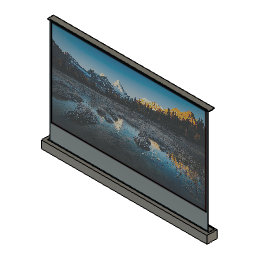
cabinet_model (Autodesk Fusion 360 archive; units mm, degrees)
design "Vividstorm S Pro 110"
Autodesk Fusion 360 part; units mm, degrees
sketch "Base sketch" plane through (0, 0, 0) normal (0, 0, 1) x (1, 0, 0)
  line L0 (0, 0) -> (2610, 0)
  line L1 (2610, 0) -> (2610, 160)
  line L2 (2610, 160) -> (0, 160)
  line L3 (0, 160) -> (0, 0)
  dimension "base_width" = 2610
  dimension "base_depth" = 160
  constraint horizontal L0
  constraint vertical L1
  constraint horizontal L2
  constraint vertical L3
  constraint coincident L0.start L3.end
  measures "base_width" distance of L0.start L0.end
  measures "base_depth" distance of L0.start L2.end
extrude "Extrude1" add sketch "Base sketch" along normal blind 120 makes body 1
sketch "Lid sketch" plane through (0, 0, 120) normal (0, 0, 1) x (-1, 0, 0)
  line L0 (0, -160) -> (0, 0)
  line L1 (0, 0) -> (-2610, 0)
  line L2 (-2610, 0) -> (-2610, -160)
  line L3 (-2610, -160) -> (0, -160)
  line L4 (-2579, -55) -> (-41, -55)
  line L5 (-41, -55) -> (-41, -150)
  line L6 (-41, -150) -> (-2579, -150)
  line L7 (-2579, -150) -> (-2579, -55)
  line L8 (0, -160) -> (0, 0)
  line L9 (0, 0) -> (-2610, 0)
  dimension "lid_width" = 2538
  dimension "lid_depth" = 95
  dimension "d51" = 41
  dimension "d52" = 55
  constraint horizontal L4
  constraint vertical L5
  constraint horizontal L6
  constraint vertical L7
  measures "lid_width" distance of L4.start L4.end
  measures "lid_depth" distance of L4.end L5.end
  measures "d51" distance of L5 L8
  measures "d52" distance of L4.end L9
extrude "Extrude2" cut sketch "Lid sketch" against normal blind 8 contours L4 L5 L6 L7 bodies 1
copy_body "Body->Comp1" bodies 1 removing the originals makes body 2 in component "Base"
sketch "Canvas sketch" plane through (0, 0, 112) normal (0, 0, 1) x (-1, 0, 0)
  line L0 (-64, -70) -> (-2553, -70)
  line L1 (-2553, -70) -> (-2553, -75)
  line L2 (-2553, -75) -> (-64, -75)
  line L3 (-64, -75) -> (-64, -70)
  line L4 (-2579, -150) -> (-41, -150)
  line L5 (-41, -150) -> (-41, -55)
  line L6 (-41, -55) -> (-2579, -55)
  line L7 (-2579, -55) -> (-2579, -150)
  dimension "d18" = 5
  dimension "d20" = 2489
  dimension "d53" = 23
  dimension "d54" = 15
  dimension "d55" = 26
  constraint horizontal L0
  constraint vertical L1
  constraint horizontal L2
  constraint vertical L3
  measures "d18" distance of L0.start L2.end
  measures "d20" distance of L0.start L0.end
  measures "d53" distance of L3 L5
  measures "d54" distance of L0 L6
  measures "d55" distance of L1.end L7
extrude "Extrude1'" add sketch "Canvas sketch" along normal blind 1650 separate body contours L0 L1 L2 L3 makes body 3 in component "Base"
copy_body "CutPasteBodies1" bodies 3 removing the originals makes body 4
copy_body "Body->Comp2" bodies 4 removing the originals makes body 5 in component "Open Canvas"
sketch "Sketch4" plane through (0, 70, 0) normal (0, -1, 0) x (1, 0, 0) in component "Open Canvas"
  line L0 (64, 112) -> (2553, 112)
  line L1 (2553, 112) -> (2553, 1762)
  line L2 (2553, 1762) -> (64, 1762)
  line L3 (64, 1762) -> (64, 112)
  line L4 (2526, 370) -> (91, 370)
  line L5 (91, 370) -> (91, 1742)
  line L6 (91, 1742) -> (2526, 1742)
  line L7 (2526, 1742) -> (2526, 370)
  dimension "d32" = 1372
  dimension "d33" = 2435
  dimension "d34" = 20
  dimension "d35" = 27
  constraint horizontal L4
  constraint vertical L5
  constraint horizontal L6
  constraint vertical L7
  measures "d32" distance of L4.start L6.end
  measures "d33" distance of L4.start L4.end
  measures "d34" distance of L2 L6
  measures "d35" distance of L3 L5
sketch "Sketch5" plane through (0, 0, 0) normal (-1, 0, 0) x (0, -1, 0)
  line L0 (-160, 0) -> (0, 0)
  line L1 (0, 0) -> (0, 120)
  line L2 (0, 120) -> (-160, 120)
  line L3 (-160, 120) -> (-160, 0)
  line L4 (-145, 52) -> (-130, 52)
  line L5 (-130, 52) -> (-130, 27)
  line L6 (-130, 27) -> (-145, 27)
  line L7 (-145, 27) -> (-145, 52)
  dimension "d36" = 15
  dimension "d37" = 27
  dimension "d38" = 15
  dimension "d39" = 25
  constraint horizontal L4
  constraint vertical L5
  constraint horizontal L6
  constraint vertical L7
  measures "d36" distance of L3 L7
  measures "d37" distance of L0 L6
  measures "d38" distance of L4.start L4.end
  measures "d39" distance of L4.end L5.end
extrude "Extrude2'" add sketch "Sketch5" along normal blind 40 contours L4 L5 L6 L7 bodies 2 in component "Base"
extrude "Extrude1''" add 1 faces at (1733, 118.3333, 112) along direction (0, 0, 1) blind 8 separate body on bodies 2 makes body 6 in component "Close Canvas"
copy_body "CopyPasteBodies2" bodies 6 makes body 7 in component "Open Canvas"
move_body "Move1" bodies 7 to x (1, 0, 0) y (0, 1, 0) z (0, 0, 1) at (0, 0, 1650) in component "Open Canvas"
combine "Combine1" operation add target body 7 tool bodies 5 in component "Open Canvas"
component "Base" placed x (1, 0, 0) y (0, 1, 0) z (0, 0, 1) at (0, 0, 0)
component "Open Canvas" placed x (1, 0, 0) y (0, 1, 0) z (0, 0, 1) at (0, 0, 0)
component "Close Canvas" placed x (1, 0, 0) y (0, 1, 0) z (0, 0, 1) at (0, 0, 0)
equation "base_height = 120 mm"
equation "d20 = viewport_vertical_offset * 2 + viewport_width"
equation "d32 = viewport_height"
equation "d33 = viewport_width"
equation "d35 = viewport_vertical_offset"
equation "cables_spacer_length = 40 mm"
equation "viewport_width = 2435.00 mm"
equation "viewport_height = 1372.00 mm"
equation "viewport_vertical_offset = 27 mm"
equation "lid_height = 8.00 mm"
equation "total_width = base_width + cables_spacer_length"
named bodies: "Canvas", "Lid"
